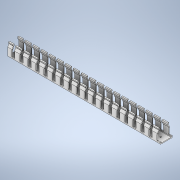
# Autodesk Inventor part: Cuerpo 30x30 378mm
Saved by Autodesk Inventor 2021 (Build 250183000, 183)
## iProperties
Created: 2021-04-16
Part Number: Cuerpo 30x30 378mm
Material: PVC, Flexible
Document SubType Name: Modeling
Designer: Nelson
Density: 1.3 g/cm^3
Appearance: PVC - White
Mass: 67.4496 g
Surface Area: 579.793 cm^2
Volume: 51.8843 cm^3
Author: Nelson
Autodesk Inventor part; units mm, degrees
ref_plane "YZ Plane" through (0, 0, 0) normal (1, 0, 0) x (0, 1, 0)
ref_plane "XZ Plane" through (0, 0, 0) normal (0, 1, 0) x (-1, 0, 0)
ref_plane "XY Plane" through (0, 0, 0) normal (0, 0, 1) x (1, 0, 0)
sketch "Boceto principal" plane through (0, 0, 0) normal (1, 0, 0) x (0, 1, 0)
  line L0 (0, -1) -> (0, -29)
  line L1 (1, -30) -> (20, -30)
  line L2 (20, -30) -> (26, -27)
  line L3 (26, -27) -> (28, -27)
  line L4 (28, -27) -> (28, -28)
  line L5 (28, -28) -> (30, -28)
  line L6 (30, -28) -> (30, -25)
  line L7 (30, -25) -> (26, -25)
  line L8 (26, -25) -> (20, -28)
  line L9 (20, -28) -> (3, -28)
  line L10 (2, -27) -> (2, -3)
  line L11 (3, -2) -> (20, -2)
  line L12 (20, -2) -> (26, -5)
  line L13 (26, -5) -> (30, -5)
  line L14 (30, -5) -> (30, -2)
  line L15 (30, -2) -> (28, -2)
  line L16 (28, -2) -> (28, -3)
  line L17 (28, -3) -> (26, -3)
  line L18 (26, -3) -> (20, 0)
  line L19 (20, 0) -> (1, 0)
  arc A0 (1, 0) -> (0, -1) centre (1, -1) ccw
  arc A1 (0, -29) -> (1, -30) centre (1, -29) ccw
  arc A2 (2, -27) -> (3, -28) centre (3, -27) ccw
  arc A3 (3, -2) -> (2, -3) centre (3, -3) ccw
  constraints: 40 end point, 8 point on circle, 4 centre point
extrude "Extrusion1" add sketch "Boceto principal" along normal blind 378
sketch "Boceto agujeros" plane through (0, 0, 0) normal (0, 0, 1) x (1, 0, 0)
  line L0 (11, 4) -> (17, 4)
  line L1 (18, 5) -> (18, 18)
  line L2 (17, 19) -> (11, 19)
  line L3 (10, 18) -> (10, 5)
  line L4 (17, 19) -> (17, 30)
  line L5 (17, 30) -> (11, 30)
  line L6 (11, 19) -> (11, 30)
  arc A0 (10, 5) -> (11, 4) centre (11, 5) ccw
  arc A1 (17, 4) -> (18, 5) centre (17, 5) ccw
  arc A2 (18, 18) -> (17, 19) centre (17, 18) ccw
  arc A3 (11, 19) -> (10, 18) centre (11, 18) ccw
  constraints: 14 end point, 8 point on circle, 4 centre point
extrude "Extrusion2" cut sketch "Boceto agujeros" against normal blind 125
pattern_linear "Rectangular Pattern1" count 23 spacing 20 along (1, 0, 0) of "Extrusion2"
sketch "Sketch3" plane through (0, 2, -3) normal (0, 1, 0) x (1, 0, 0)
  line L0 (0, 24) -> (0, 0) projected
  line L1 (378, 24) -> (378, 0) projected
  line L2 (17, 27) -> (31, 27) projected
  line L3 (197, 27) -> (211, 27) projected
  line L4 (337, 27) -> (351, 27) projected
  point P0 (0, -3)
  point P1 (14, 12)
  point P2 (189, 12)
  point P3 (364, 12)
  dimension "d7" = 14
  dimension "d8" = 14
  dimension "d9" = 189
  dimension "d10" = 15
  dimension "d11" = 15
  dimension "d12" = 15
  measures "d7" distance from line of point (14, 12) L0
  measures "d8" distance from line of L1 point (364, 12)
  measures "d9" distance from line of point (189, 12) L0
  measures "d10" distance from line of point (14, 12) L2
  measures "d11" distance from line of L3 point (189, 12)
  measures "d12" distance from line of L4 point (364, 12)
hole "Hole1" at (14, 2, -15) at (189, 2, -15) at (364, 2, -15) direction (0, -1, 0) diameter 3.8 depth 8 tip angle 118
sketch "Sketch4" plane through (378, 0, 0) normal (1, 0, 0) x (0, 0, -1)
  line L0 (-4.3359, 32.9222) -> (35.1117, 32.9222)
  line L1 (35.1117, 32.9222) -> (35.1117, 15.481)
  line L2 (35.1117, 15.481) -> (-4.3359, 15.481)
  line L3 (-4.3359, 15.481) -> (-4.3359, 32.9222)
  point P0 (0, 0)
  constraints: 8 end point, 2 parallel, 1 horizontal, 1 perpendicular
extrude "Extrusion3" cut sketch "Sketch4" against normal blind 3
equation "\"d8\" = d7"
equation "\"d11\" = d10"
equation "\"d12\" = d10"
body "Solid1"
